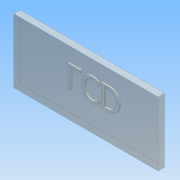
# Autodesk Inventor part: LCD
Saved by Autodesk Inventor 2016 (Build 200138000, 138)
## iProperties
Created: 2016-04-03
Part Number: LCD
Material: Glass
Document SubType Name: Modeling
Designer: admin
Density: 2.18 g/cm^3
Appearance: Clear
Author: admin
Autodesk Inventor part; units mm, degrees
ref_plane "YZ Plane" through (0, 0, 0) normal (1, 0, 0) x (0, 1, 0)
ref_plane "XZ Plane" through (0, 0, 0) normal (0, 1, 0) x (-1, 0, 0)
ref_plane "XY Plane" through (0, 0, 0) normal (0, 0, 1) x (1, 0, 0)
sketch "Sketch1" plane through (0, 0, 0) normal (0, 1, 0) x (-1, 0, 0)
  line L0 (22.5, -10) -> (-22.5, -10)
  line L1 (-22.5, -10) -> (-22.5, 10)
  line L2 (-22.5, 10) -> (22.5, 10)
  line L3 (22.5, 10) -> (22.5, -10)
  point P0 (0, 0)
  point P1 (22.5, 0)
  point P2 (0, -10)
  dimension "d0" = 45
  dimension "d1" = 20
  constraints: 8 end point, 2 midpoint, 2 parallel, 1 horizontal, 1 horizontal alignment, 1 perpendicular, 1 vertical alignment
  measures "d0" distance of L0.start L0.end
  measures "d1" distance of L2.end L0.start
extrude "Extrusion1" add sketch "Sketch1" along normal blind 2
sketch "Sketch2" plane through (0, 2, 0) normal (0, 1, 0) x (1, 0, 0)
  line L0 (-8.5073, 4.0617) -> (8.5899, 4.0617) construction
  line L1 (8.5899, 4.0617) -> (8.5899, -3.1879) construction
  line L2 (8.5899, -3.1879) -> (-8.5073, -3.1879) construction
  line L3 (-8.5073, -3.1879) -> (-8.5073, 4.0617) construction
  line L4 (-3.7423, -3.0631) -> (-7.7982, -3.0631)
  line L5 (-7.7982, -3.0631) -> (-7.7982, 3.9369)
  line L6 (-7.7982, 3.9369) -> (-6.8679, 3.9369)
  line L7 (-6.8679, 3.9369) -> (-6.8679, -2.2349)
  line L8 (-6.8679, -2.2349) -> (-3.7423, -2.2349)
  line L9 (-3.7423, -2.2349) -> (-3.7423, -3.0631)
  spline S0 degree 2 poles (-0.2764, -3.1879) (-0.9571, -3.1879) (-2.1086, -2.7284) (-2.5284, -2.2689) knots 0 0 0 1 2 2 2
  spline S1 degree 2 poles (-2.5284, -2.2689) (-2.9482, -1.8151) (-3.4076, -0.4537) (-3.4076, 0.4312) knots 0 0 0 1 2 2 2
  spline S2 degree 2 poles (-3.4076, 0.4312) (-3.4076, 1.3105) (-2.9595, 2.6152) (-2.5341, 3.0973) knots 0 0 0 1 2 2 2
  spline S3 degree 2 poles (-2.5341, 3.0973) (-2.1143, 3.5682) (-0.9684, 4.0617) (-0.2593, 4.0617) knots 0 0 0 1 2 2 2
  spline S4 degree 2 poles (-0.2593, 4.0617) (0.0924, 4.0617) (0.7107, 3.9596) (0.9716, 3.8802) knots 0 0 0 1 2 2 2
  spline S5 degree 2 poles (0.9716, 3.8802) (1.1985, 3.8064) (1.6693, 3.5965) (1.9019, 3.4717) knots 0 0 0 1 2 2 2
  line L10 (1.9019, 3.4717) -> (1.9019, 2.3486)
  line L11 (1.9019, 2.3486) -> (1.8282, 2.3486)
  spline S6 degree 2 poles (1.8282, 2.3486) (1.7034, 2.462) (1.3176, 2.7797) (1.0397, 2.9328) knots 0 0 0 1 2 2 2
  spline S7 degree 2 poles (1.0397, 2.9328) (0.7731, 3.0803) (0.1434, 3.2675) (-0.265, 3.2675) knots 0 0 0 1 2 2 2
  spline S8 degree 2 poles (-0.265, 3.2675) (-0.7132, 3.2675) (-1.513, 2.8988) (-1.8136, 2.5471) knots 0 0 0 1 2 2 2
  spline S9 degree 2 poles (-1.8136, 2.5471) (-2.1086, 2.1897) (-2.4376, 1.1063) (-2.4376, 0.4312) knots 0 0 0 1 2 2 2
  spline S10 degree 2 poles (-2.4376, 0.4312) (-2.4376, -0.2892) (-2.0916, -1.3273) (-1.791, -1.6847) knots 0 0 0 1 2 2 2
  spline S11 degree 2 poles (-1.791, -1.6847) (-1.496, -2.0307) (-0.7075, -2.3824) (-0.265, -2.3824) knots 0 0 0 1 2 2 2
  spline S12 degree 2 poles (-0.265, -2.3824) (0.1377, -2.3824) (0.8241, -2.1839) (1.0907, -2.0364) knots 0 0 0 1 2 2 2
  spline S13 degree 2 poles (1.0907, -2.0364) (1.346, -1.8889) (1.7261, -1.5826) (1.8338, -1.4748) knots 0 0 0 1 2 2 2
  line L12 (1.8338, -1.4748) -> (1.9019, -1.4748)
  line L13 (1.9019, -1.4748) -> (1.9019, -2.5866)
  spline S14 degree 2 poles (1.9019, -2.5866) (1.6693, -2.6944) (1.2609, -2.8929) (0.9716, -2.9837) knots 0 0 0 1 2 2 2
  spline S15 degree 2 poles (0.9716, -2.9837) (0.6653, -3.0858) (0.1434, -3.1879) (-0.2764, -3.1879) knots 0 0 0 1 2 2 2
  spline S16 degree 2 poles (8.2893, 0.4312) (8.2893, -0.5274) (7.5121, -2.0704) (6.8598, -2.5015) knots 0 0 0 1 2 2 2
  spline S17 degree 2 poles (6.8598, -2.5015) (6.3265, -2.8362) (5.2317, -3.0631) (4.3808, -3.0631) knots 0 0 0 1 2 2 2
  line L14 (4.3808, -3.0631) -> (2.7698, -3.0631)
  line L15 (2.7698, -3.0631) -> (2.7698, 3.9369)
  line L16 (2.7698, 3.9369) -> (4.3638, 3.9369)
  spline S18 degree 2 poles (4.3638, 3.9369) (5.3509, 3.9369) (6.474, 3.6419) (6.8711, 3.381) knots 0 0 0 1 2 2 2
  spline S19 degree 2 poles (6.8711, 3.381) (7.5462, 2.9328) (8.2893, 1.4523) (8.2893, 0.4312) knots 0 0 0 1 2 2 2
  spline S20 degree 2 poles (7.3193, 0.4426) (7.3193, 1.2481) (6.786, 2.3883) (6.2585, 2.7116) knots 0 0 0 1 2 2 2
  spline S21 degree 2 poles (6.2585, 2.7116) (5.8841, 2.9328) (5.0389, 3.1314) (4.4092, 3.1314) knots 0 0 0 1 2 2 2
  line L17 (4.4092, 3.1314) -> (3.7001, 3.1314)
  line L18 (3.7001, 3.1314) -> (3.7001, -2.2576)
  line L19 (3.7001, -2.2576) -> (4.4092, -2.2576)
  spline S22 degree 2 poles (4.4092, -2.2576) (5.0275, -2.2576) (5.9635, -2.0591) (6.3436, -1.7924) knots 0 0 0 1 2 2 2
  spline S23 degree 2 poles (6.3436, -1.7924) (6.8314, -1.4634) (7.3193, -0.3743) (7.3193, 0.4426) knots 0 0 0 1 2 2 2
  point P0 (0, 0)
  constraints: 2 other
emboss "Emboss1" sketch "Sketch2" operation add depth 0.5 direction (0, -1, 0)
body "Solid1"
